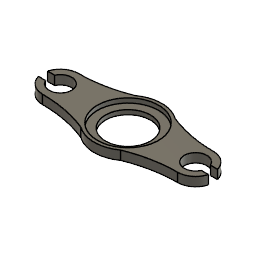
Exercise_7_Problem (Autodesk Fusion 360 design; units mm, degrees)
part number: 2026-05-20-10-56-49-003
Autodesk Fusion 360 part; units mm, degrees
sketch "Sketch1" plane through (0, 0, 0) normal (0, 1, 0) x (1, 0, 0)
  line L0 (190, -75) -> (-190, -75)
  line L1 (-190, -75) -> (-190, 75)
  line L2 (-190, 75) -> (190, 75)
  line L3 (190, 75) -> (190, -75)
  line L4 (190, -75) -> (-190, 75) construction
  line L5 (-190, -75) -> (190, 75) construction
  dimension "d1" = 380
  dimension "d2" = 150
  constraint horizontal L0
  constraint perpendicular L0 L1
  constraint parallel L0 L2
  constraint parallel L1 L3
  constraint coincident L4 origin
  constraint coincident L5 origin
  measures "d1" distance of L1.end L2.end
  measures "d2" distance of L0.end L1.end
extrude "Extrude1" add sketch "Sketch1" along normal blind 20
sketch "Sketch2" plane through (0, 20, 0) normal (0, 1, 0) x (-1, 0, 0)
  line L0 (-190, -75) -> (190, -75)
  line L1 (190, -75) -> (190, 75)
  line L2 (190, 75) -> (-190, 75)
  line L3 (-190, 75) -> (-190, -75)
  circle A0 centre (0, 0) radius 75
  line L4 (0, 0) -> (-150, 0)
  line L5 (0, 0) -> (150, 0)
  circle A1 centre (150, 0) radius 40
  circle A2 centre (-150, 0) radius 40
  line L6 (190, 0) -> (175, 0)
  line L7 (175, 0) -> (175, -10)
  line L8 (175, -10) -> (188.7298, -10)
  line L9 (175, 0) -> (175, 10)
  line L10 (175, 10) -> (188.7298, 10)
  line L11 (-190, 0) -> (-175, 0)
  line L12 (-175, 0) -> (-175, -10)
  line L13 (-175, 0) -> (-175, 10)
  line L14 (-175, -10) -> (-188.7298, -10)
  line L15 (-175, 10) -> (-188.7298, 10)
  line L16 (-188.7298, -10) -> (-190, -10)
  line L17 (-188.7298, 10) -> (-190, 10)
  line L18 (188.7298, -10) -> (190, -10)
  line L19 (188.7298, 10) -> (190, 10)
  circle A3 centre (150, 0) radius 25
  line L20 (175, -10) -> (172.9129, -10)
  line L21 (172.9129, 10) -> (175, 10)
  line L22 (172.9129, 10) -> (172.9129, -10)
  circle A4 centre (-150, 0) radius 25
  line L23 (-175, -10) -> (-172.9129, -10)
  line L24 (-172.9129, -10) -> (-172.9129, 10)
  line L25 (-172.9129, 10) -> (-175, 10)
  line L26 (-190, 10) -> (-190, -10)
  line L27 (-188.7298, -10) -> (-190, -10)
  line L28 (-188.7298, 10) -> (-190, 10)
  line L29 (0, -75) -> (-190, -75)
  line L30 (0, -75) -> (0, 75)
  line L31 (-190, 75) -> (-190, -75)
  line L32 (-150, 0) -> (-150, -75)
  line L33 (-150, 0) -> (-150, 75)
  line L34 (0, 75) -> (-150, 75)
  line L35 (150, 0) -> (150, 75)
  line L36 (0, 75) -> (150, 75)
  line L37 (150, 0) -> (150, -75)
  line L38 (150, -75) -> (0, -75)
  arc A5 (150, -40) -> (44.1171, -60.6521) centre (150, -321.7554) ccw
  arc A6 (-44.1171, -60.6521) -> (-150, -40) centre (-150, -321.7554) ccw
  arc A7 (-150, 40) -> (-44.1171, 60.6521) centre (-150, 321.7554) ccw
  arc A8 (44.1171, 60.6521) -> (150, 40) centre (150, 321.7554) ccw
  dimension "d5" = 150
  dimension "d6" = 150
  dimension "d7" = 80
  dimension "d19" = 15
  dimension "d20" = 10
  dimension "d21" = 10
  dimension "d22" = 15
  dimension "d23" = 10
  dimension "d24" = 10
  constraint coincident A0.centre L4.start
  constraint horizontal L4
  constraint parallel L4 L5
  constraint coincident L5.end A1.centre
  constraint coincident L4.end A2.centre
  constraint midpoint L1 L6.start
  constraint perpendicular L1 L6
  constraint perpendicular L6 L7
  constraint coincident A1 L8.end
  constraint perpendicular L1 L8
  constraint perpendicular L6 L9
  constraint coincident A1 L10.end
  constraint perpendicular L1 L10
  constraint midpoint L3 L11.start
  constraint perpendicular L3 L11
  constraint perpendicular L11 L12
  constraint perpendicular L11 L13
  constraint coincident A2 L14.end
  constraint perpendicular L3 L14
  constraint coincident A2 L15.end
  constraint perpendicular L3 L15
  constraint coincident L3 L16.end
  constraint perpendicular L3 L16
  constraint coincident L3 L17.end
  constraint perpendicular L3 L17
  constraint coincident L1 L18.end
  constraint perpendicular L1 L18
  constraint coincident L1 L19.end
  constraint perpendicular L1 L19
  constraint concentric A1 A3
  constraint coincident A3 L20.end
  constraint perpendicular L7 L20
  constraint coincident A3 L21.start
  constraint perpendicular L9 L21
  constraint concentric A2 A4
  constraint coincident L11.end A4
  constraint coincident A4 L23.end
  constraint perpendicular L12 L23
  constraint coincident A4 L24.end
  constraint perpendicular L23 L24
  constraint midpoint L0 L29.start
  constraint coincident L0.start L3.end
  constraint midpoint L2 L30.end
  constraint coincident L2.end L3.start
  constraint coincident L29 L32.end
  constraint coincident L2 L33.end
  constraint perpendicular L2 L33
  constraint coincident L2 L35.end
  constraint perpendicular L2 L35
  constraint coincident L0 L37.end
  constraint perpendicular L0 L37
  constraint coincident L32 A6.end
  constraint coincident A2 A6.end
  constraint coincident A2 A7.start
  constraint coincident L33 A7.start
  constraint coincident A1 A8.end
  constraint coincident L35 A8.end
  constraint coincident L37 A5.start
  constraint coincident A1 A5.start
  constraint tangent A1 A5
  constraint tangent A2 A6
  constraint tangent A2 A7
  constraint tangent A1 A8
  constraint coincident A0 A5.end
  constraint coincident A0 A6.start
  constraint coincident A0 A7.end
  constraint coincident A0 A8.start
  measures "d5" diameter of A0
  measures "d6" distance of A0.centre L5.end
  measures "d7" diameter of A1
  measures "d19" distance of L6.start L6.end
  measures "d20" distance of L6.end L7.end
  measures "d21" distance of L6.end L9.end
  measures "d22" distance of L11.start L11.end
  measures "d23" distance of L11.end L12.end
  measures "d24" distance of L11.end L13.end
hole "Hole1" at (0, 20, 0) direction (0, -1, 0) diameter 100 depth 20 tip angle 180 counterbore diameter 135.6 counterbore depth 10
hole "Hole2" at (-150, 20, 0) direction (0, -1, 0) diameter 50 depth 20 tip angle 180
hole "Hole3" at (150, 20, 0) direction (0, -1, 0) diameter 50 depth 20 tip angle 180
extrude "Extrude2" cut sketch "Sketch2" against normal blind 20 contours A2 L11 L12 L14 | A2 L11 L13 L15 | A1 L6 L7 L8 | A1 L6 L9 L10
extrude "Extrude3" cut sketch "Sketch2" against normal blind 20 contours L1 A1 L18 | L1 A1 L19
extrude "Extrude4" cut sketch "Sketch2" against normal blind 20 contours L7 A3 L20 | L9 A3 L21
extrude "Extrude5" cut sketch "Sketch2" against normal blind 20 contours L12 A4 L23 | L13 A4 L25
extrude "Extrude6" cut sketch "Sketch2" against normal blind 20 contours L3 A2 L16 L26 L27 L31 | L3 A2 L17 L26 L28 L31
extrude "Extrude7" cut sketch "Sketch2" against normal blind 20 contours L0 L3 A2 L16 L27 L29 L31 L32 | L0 A0 L29 L32 A6 | L0 A0 L37 L38 A5 | L0 L1 A1 L18 L37 | L2 L3 A2 L17 L28 L31 L33 | L2 A0 L33 L34 A7 | L2 A0 L35 L36 A8 | L1 L2 A1 L19 L35
